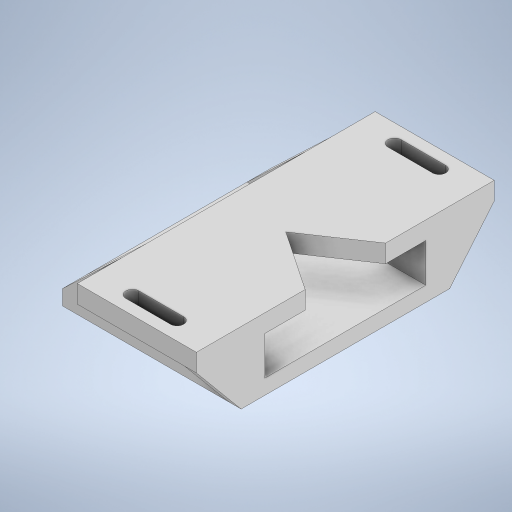
# Autodesk Inventor part: soporte infe
Saved by Autodesk Inventor 2024 (Build 280153000, 153)
## iProperties
Created: 2024-04-18
Part Number: soporte infe
Material: Generic
Document SubType Name: Modeling
Designer: compu
Density: 1 g/cm^3
Appearance: Default
Author: compu
Autodesk Inventor part; units mm, degrees
ref_plane "YZ Plane" through (0, 0, 0) normal (1, 0, 0) x (0, 1, 0)
ref_plane "XZ Plane" through (0, 0, 0) normal (0, 1, 0) x (-1, 0, 0)
ref_plane "XY Plane" through (0, 0, 0) normal (0, 0, 1) x (1, 0, 0)
sketch "Sketch1" plane through (0, 0, 0) normal (0, 1, 0) x (-1, 0, 0)
  line L0 (8, 0) -> (-48, 0) projected
  line L1 (0, -70) -> (0, 70) projected
  line L2 (-40, 50) -> (0, 50)
  line L3 (0, 50) -> (0, -50)
  line L4 (0, -50) -> (-40, -50)
  line L5 (-40, -50) -> (-40, 50)
  point P0 (0, 0)
  point P1 (0, 50)
  dimension "d0" = 40
  dimension "d1" = 100
  constraints: 8 end point, 2 parallel, 1 collinear, 1 horizontal, 1 perpendicular, 1 other
  measures "d0" distance of L3.end L4.end
  measures "d1" distance of L2.end L3.end
extrude "Extrusion1" add sketch "Sketch1" against normal blind 6
sketch "Sketch2" plane through (0, -6, 0) normal (0, -1, 0) x (1, 0, 0)
  line L0 (0, -50) -> (40, -50) projected
  line L1 (40, -50) -> (40, 50) projected
  line L2 (40, 50) -> (0, 50) projected
  line L3 (0, 50) -> (0, -50) projected
  line L4 (40, 35) -> (0, 35)
  line L5 (40, -50) -> (40, 50) projected
  line L6 (40, -35) -> (0, -35)
  line L7 (40, 27) -> (0, 27)
  line L8 (40, -27) -> (0, -27)
  point P0 (0, 0)
  dimension "d4" = 15
  dimension "d5" = 15
  dimension "d6" = 8
  dimension "d7" = 8
  constraints: 8 end point, 8 point on line, 4 perpendicular
  measures "d4" distance between parallel lines of L2 L4
  measures "d5" distance between parallel lines of L0 L6
  measures "d6" distance between parallel lines of L4 L7
  measures "d7" distance between parallel lines of L6 L8
extrude "Extrusion2" add sketch "Sketch2" along normal blind 18 contours L3 L8 L1 L6 | L3 L4 L1 L7
sketch "Sketch3" plane through (0, 0, 0) normal (0, 1, 0) x (1, 0, 0)
  line L0 (40, 50) -> (0, 50) projected
  line L1 (0, 50) -> (0, -50) projected
  line L2 (0, -50) -> (40, -50) projected
  line L3 (40, -50) -> (40, 50) projected
  line L4 (0, -44) -> (40, -44) construction
  arc A0 (12.5, -41.8) -> (12.5, -46.2) centre (12.5, -44) ccw
  arc A1 (27.5, -46.2) -> (27.5, -41.8) centre (27.5, -44) ccw
  line L5 (12.5, -41.8) -> (27.5, -41.8)
  line L6 (12.5, -46.2) -> (27.5, -46.2)
  line L7 (-8, 0) -> (48, 0) projected
  arc A2 (12.5, 46.2) -> (12.5, 41.8) centre (12.5, 44) ccw
  arc A3 (27.5, 41.8) -> (27.5, 46.2) centre (27.5, 44) ccw
  line L8 (12.5, 41.8) -> (27.5, 41.8)
  line L9 (12.5, 46.2) -> (27.5, 46.2)
  point P0 (0, 0)
  dimension "d10" = 6
  dimension "d11" = 4.4
  dimension "d12" = 4.4
  dimension "d13" = 15
  dimension "d14" = 12.5
  constraints: 10 end point, 8 point on circle, 6 symmetric about line, 4 centre point, 4 point on line, 2 horizontal, 2 tangent, 1 perpendicular, 2 other
  measures "d10" distance between parallel lines of L2 L4
  measures "d11" diameter of A0
  measures "d12" diameter of A1
  measures "d13" distance of A1.centre A0.centre
  measures "d14" distance from line of L3 A1.centre
extrude "Extrusion3" cut sketch "Sketch3" against normal blind 18 contours L5 A1 L6 A0 | L9 A3 L8 A2
sketch "Sketch4" plane through (0, -24, 0) normal (0, -1, 0) x (1, 0, 0)
  line L0 (40, 35) -> (-20, 35)
  line L1 (-20, 35) -> (-20, -35)
  line L2 (-20, -35) -> (40, -35)
  line L3 (40, -35) -> (40, 35)
  line L4 (40, 27) -> (40, 35) projected
  line L5 (40, 35) -> (0, 35) projected
  line L6 (0, 35) -> (0, 27) projected
  line L7 (0, 27) -> (40, 27) projected
  line L8 (0, -27) -> (0, -35) projected
  line L9 (0, -35) -> (40, -35) projected
  line L10 (40, -35) -> (40, -27) projected
  line L11 (40, -27) -> (0, -27) projected
  line L12 (40, 35) -> (0, 35) projected
  line L13 (0, -35) -> (40, -35) projected
  line L14 (40, -27) -> (40, 27) projected
  line L15 (40, -35) -> (40, -27) projected
  point P0 (0, 0)
  dimension "d18" = 20
  constraints: 8 end point, 3 collinear, 2 parallel, 1 horizontal, 1 perpendicular
  measures "d18" distance between parallel lines of L8 L1
extrude "Extrusion4" add sketch "Sketch4" against normal blind 5
sketch "Sketch5" plane through (0, 0, 0) normal (0, 1, 0) x (1, 0, 0)
  arc A0 (27.5, 41.8) -> (27.5, 46.2) centre (27.5, 44) ccw projected
  line L0 (27.5, 41.8) -> (12.5, 41.8) projected
  arc A1 (12.5, 46.2) -> (12.5, 41.8) centre (12.5, 44) ccw projected
  line L1 (12.5, 46.2) -> (27.5, 46.2) projected
  arc A2 (27.5, -46.2) -> (27.5, -41.8) centre (27.5, -44) ccw projected
  line L2 (27.5, -46.2) -> (12.5, -46.2) projected
  arc A3 (12.5, -41.8) -> (12.5, -46.2) centre (12.5, -44) ccw projected
  line L3 (12.5, -41.8) -> (27.5, -41.8) projected
  line L4 (40, 50) -> (0, 50) projected
  line L5 (0, 50) -> (0, -50) projected
  line L6 (0, -50) -> (40, -50) projected
  line L7 (40, -50) -> (40, 50) projected
  line L8 (-32, 0) -> (52, 0) projected
  line L9 (40, -27) -> (0, -27) projected
  line L10 (0, 27) -> (40, 27) projected
  line L11 (40, -27) -> (40, 0) construction
  line L12 (40, 27) -> (40, 0) construction
  line L13 (40, -13.5) -> (20, 0)
  line L14 (20, 0) -> (40, 13.5)
  line L15 (40, -13.5) -> (46.5752, -13.5)
  line L16 (46.5752, -13.5) -> (46.5752, 13.5)
  line L17 (46.5752, 13.5) -> (40, 13.5)
  point P0 (0, 0)
  dimension "d21" = 20
  constraints: 14 end point, 3 midpoint, 3 perpendicular, 2 point on line, 1 horizontal
  measures "d21" distance from line of L5 L13.end
extrude "Extrusion5" cut sketch "Sketch5" against normal up to surface (19 mm away) contours L17 L16 L8 L7 | L7 L8 L14 | L8 L16 L15 L7 | L7 L13 L8
sketch "Sketch6" plane through (40, -6, 50) normal (1, 0, 0) x (0, 0, -1)
  line L0 (36.5, 0) -> (36.5, 6) projected
  line L1 (0, 6) -> (36.5, 6) projected
  line L2 (0, 6) -> (0, 0) projected
  line L3 (15, 0) -> (0, 0) projected
  line L4 (15, 0) -> (15, -18) projected
  line L5 (85, -18) -> (15, -18) projected
  line L6 (85, 0) -> (85, -18) projected
  line L7 (100, 0) -> (85, 0) projected
  line L8 (100, 6) -> (100, 0) projected
  line L9 (63.5, 6) -> (100, 6) projected
  line L10 (63.5, 6) -> (63.5, 0) projected
  line L11 (77, 0) -> (63.5, 0) projected
  line L12 (77, 0) -> (77, -13) projected
  line L13 (23, -13) -> (77, -13) projected
  line L14 (23, 0) -> (23, -13) projected
  line L15 (36.5, 0) -> (23, 0) projected
  line L16 (100, 0) -> (85, -18)
  line L17 (85, 0) -> (85, -18)
  line L18 (100, 0) -> (85, 0)
  line L19 (0, 0) -> (15, 0)
  line L20 (3.8, 6) -> (3.8, 0) projected
  line L21 (15, -18) -> (15, 0)
  line L22 (0, 0) -> (15, -18)
  point P0 (50, 6)
  constraints: 12 end point, 2 collinear, 2 perpendicular
extrude "Extrusion6" add sketch "Sketch6" against normal blind 4 contours L3 L4 L22 | L6 L7 L16
sketch "Sketch7" plane through (-20, -19, 35) normal (0, 0, 1) x (1, 0, 0)
  line L0 (20, 19) -> (60, 19) projected
  line L1 (20, 19) -> (20, 13) projected
  line L2 (56, 13) -> (20, 13) projected
  line L3 (60, 13) -> (56, 13) projected
  line L4 (60, 19) -> (60, 13) projected
  line L5 (56, -5) -> (56, 13) projected
  line L6 (20, 13) -> (56, 13) projected
  line L7 (20, 13) -> (20, 0) projected
  line L8 (0, 0) -> (20, 0) projected
  line L9 (0, -5) -> (0, 0) projected
  line L10 (56, -5) -> (0, -5) projected
  line L11 (60, 19) -> (20, 19) projected
  line L12 (20, 19) -> (0, 0)
  line L13 (20, 0) -> (20, 19)
  line L14 (0, 0) -> (20, 0)
  constraints: 6 end point, 1 collinear, 1 perpendicular
extrude "Extrusion7" add sketch "Sketch7" against normal blind 8 contours L1 L7 L8 L12
sketch "Sketch8" plane through (0, -19, -35) normal (0, 0, -1) x (-1, 0, 0)
  line L0 (0, 19) -> (-40, 19) projected
  line L1 (0, 19) -> (0, 13) projected
  line L2 (-36, 13) -> (0, 13) projected
  line L3 (-40, 13) -> (-36, 13) projected
  line L4 (-40, 19) -> (-40, 13) projected
  line L5 (-36, -5) -> (-36, 13) projected
  line L6 (0, 13) -> (-36, 13) projected
  line L7 (0, 19) -> (0, 13) projected
  line L8 (0, 19) -> (20, 0) projected
  line L9 (20, -5) -> (20, 0) projected
  line L10 (-36, -5) -> (20, -5) projected
  line L11 (0, 19) -> (20, 0)
  line L12 (20, 0) -> (-40, 0) projected
  line L13 (0, 0) -> (0, 19)
  line L14 (20, 0) -> (0, 0)
  point P0 (0, 19)
  constraints: 6 end point, 2 collinear, 1 point on line
extrude "Extrusion8" add sketch "Sketch8" against normal blind 8 contours L8 L12 L13 L1
body "Solid1"
